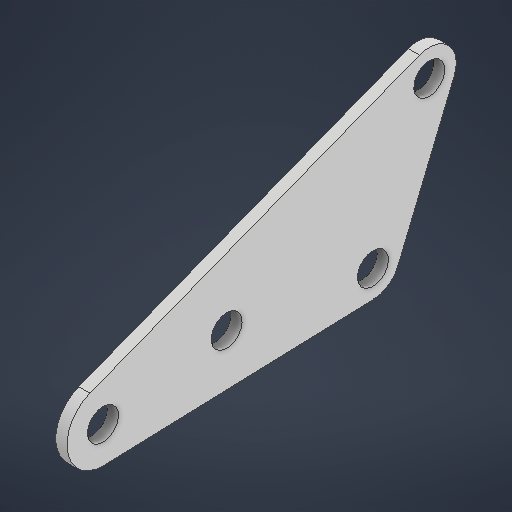
# Autodesk Inventor part: rotationmount
Saved by Autodesk Inventor 2025.2 (Build 292293000, 293)
## iProperties
Created: 2025-04-17
Part Number: rotationmount
Material: Generic
Document SubType Name: Modeling
Designer: roejo
Density: 1 g/cm^3
Appearance: Default
Author: roejo
Autodesk Inventor part; units mm, degrees
ref_plane "YZ Plane" through (0, 0, 0) normal (1, 0, 0) x (0, 1, 0)
ref_plane "XZ Plane" through (0, 0, 0) normal (0, 1, 0) x (-1, 0, 0)
ref_plane "XY Plane" through (0, 0, 0) normal (0, 0, 1) x (1, 0, 0)
sketch "Sketch1" plane through (0, 0, 0) normal (1, 0, 0) x (0, 1, 0)
  circle A0 centre (0, 0) radius 2.1844
  circle A1 centre (0, 0) radius 3.81
  circle A2 centre (0.0028, 38.1001) radius 2.1844
  circle A3 centre (0.0028, 38.1001) radius 5.08
  line L0 (0, 0) -> (16.51, 0) construction
  circle A4 centre (19.2535, -7.9481) radius 2.1844
  line L1 (0, 0) -> (16.51, 0) construction
  circle A5 centre (2.7435, 20.6481) radius 2.1844
  circle A6 centre (2.7435, 20.6481) radius 3.81
  circle A7 centre (19.2535, -7.9481) radius 3.81
  line L2 (0, 0) -> (12.7, 0) construction
  line L3 (-5.0744, 37.9311) -> (-3.8079, -0.1267)
  line L4 (-1.4538, -3.5217) -> (17.7997, -11.4698)
  line L5 (4.7381, 39.9396) -> (22.805, -6.5685)
  dimension "d0" = 4.3688
  dimension "d1" = 7.62
  dimension "d3" = 4.3688
  dimension "d4" = 10.16
  dimension "d8" = 4.3688
  dimension "d11" = 4.3688
  dimension "d12" = 7.62
  dimension "d13" = 7.62
  constraints: 12 end point, 8 centre point, 6 point on circle, 6 tangent, 5 coincident, 3 horizontal
  measures "d0" diameter of A0
  measures "d1" diameter of A1
  measures "d3" diameter of A2
  measures "d4" diameter of A3
  measures "d8" diameter of A4
  measures "d11" diameter of A5
  measures "d12" diameter of A6
  measures "d13" diameter of A7
extrude "Extrusion1" add sketch "Sketch1" along normal blind 1.5875 contours A1 | A1 L3 A3 L5 A7 L4 | A3 | A7 | A6
body "Solid1"
